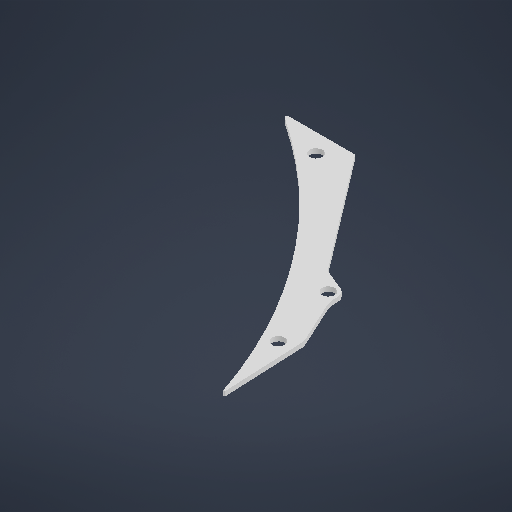
# Autodesk Inventor part: ramptest
Saved by Autodesk Inventor 2025.2 (Build 292293000, 293)
## iProperties
Created: 2025-04-12
Part Number: ramptest
Material: Generic
Document SubType Name: Modeling
Designer: Jahan
Density: 1 g/cm^3
Appearance: Default
Author: Jahan
Autodesk Inventor part; units mm, degrees
ref_plane "YZ Plane" through (0, 0, 0) normal (1, 0, 0) x (0, 1, 0)
ref_plane "XZ Plane" through (0, 0, 0) normal (0, 1, 0) x (-1, 0, 0)
ref_plane "XY Plane" through (0, 0, 0) normal (0, 0, 1) x (1, 0, 0)
sketch "Sketch1" plane through (0, 0, 0) normal (0, 1, 0) x (-1, 0, 0)
  line L0 (-8.6783, 63.9266) -> (-7.4672, 37.0366)
  arc A0 (-7.4665, 37.0351) -> (-7.2437, 35.3675) centre (-1.1165, 37.0351) ccw
  arc A1 (-8.0603, 64.0426) -> (-8.6783, 63.9266) centre (-8.3611, 63.9409) ccw
  circle A2 centre (46.3644, -22.1415) radius 2.1844
  circle A3 centre (-3.0025, 40.1702) radius 2.1844
  circle A4 centre (3.2141, 16.7955) radius 2.1844
  arc A5 (61.9811, -28.4915) -> (62.3312, -27.3267) centre (61.9811, -27.8565) ccw
  arc A6 (-8.0603, 64.0426) -> (62.3312, -27.3267) centre (160.3691, 121.002) ccw
  line L1 (3.2141, 16.7955) -> (7.9766, 16.7955) construction
  line L2 (-0.9427, 21.666) -> (-7.2437, 35.3675)
  arc A7 (0.0392, 16.7937) -> (-0.9427, 21.666) centre (-10.7551, 17.1535) ccw
  arc A8 (0.0392, 16.7937) -> (3.2141, 13.6205) centre (3.1101, 16.6914) ccw
  arc A9 (39.2923, -28.4027) -> (39.6161, -28.4915) centre (39.6161, -27.8565) ccw
  line L3 (61.9811, -28.4915) -> (39.6161, -28.4915)
  line L4 (1.9543, 13.8444) -> (9.4601, 10.7972)
  line L5 (9.4601, 10.7972) -> (39.2923, -28.4027)
  point P0 (0, 0)
  dimension "d5" = 4.3688
  dimension "d9" = 4.3688
  dimension "d10" = 4.3688
  dimension "d12" = 0.635
  dimension "d26" = 0.635
  constraints: 15 point on circle, 12 end point, 10 centre point, 4 tangent, 2 horizontal, 1 other
  measures "d5" diameter of A2
  measures "d9" diameter of A3
  measures "d10" diameter of A4
  measures "d12" radius of A5
  measures "d26" radius of A9
extrude "Extrusion2" add sketch "Sketch1" along normal blind 1.5875
body "Solid2"
